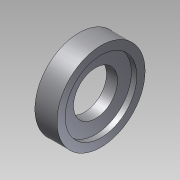
# Autodesk Inventor part: Pusher.springplate
Saved by Autodesk Inventor 2011 (Build 150239000, 239)
## iProperties
Created: 2011-04-01
Part Number: Pusher.springplate
Document SubType Name: Modeling
Designer: Casey
Density: 1 g/cm^3
Author: Casey
Autodesk Inventor part; units mm, degrees
ref_plane "YZ Plane" through (0, 0, 0) normal (1, 0, 0) x (0, 1, 0)
ref_plane "XZ Plane" through (0, 0, 0) normal (0, 1, 0) x (-1, 0, 0)
ref_plane "XY Plane" through (0, 0, 0) normal (0, 0, 1) x (1, 0, 0)
sketch "Sketch1" plane through (0, 0, 0) normal (0, 0, 1) x (1, 0, 0)
  line L0 (0, 2) -> (0.5, 2)
  line L1 (0.5, 2) -> (0.5, 3.25)
  line L2 (0.5, 3.25) -> (1, 3.25)
  line L3 (1, 3.25) -> (1, 4)
  line L4 (1, 4) -> (0, 4)
  line L5 (0, 4) -> (0, 2) construction
  line L6 (0, 0) -> (5.2426, 0) construction
  line L7 (0, 2) -> (-0.5, 2)
  line L8 (-0.5, 2) -> (-0.5, 3.25)
  line L9 (-0.5, 3.25) -> (-1, 3.25)
  line L10 (-1, 3.25) -> (-1, 4)
  line L11 (-1, 4) -> (0, 4)
  dimension "d0" = 4
  dimension "d1" = 0.5
  dimension "d2" = 8
  dimension "d4" = 0.5
  dimension "d5" = 6.5
  constraints: 24 end point, 4 symmetric about line, 3 parallel, 3 perpendicular, 1 horizontal, 1 point on line
  measures "d0" diameter of L0 L6
  measures "d1" distance between parallel lines of L3 L1
  measures "d2" diameter of L4 L6
  measures "d4" distance between parallel lines of L5 L1
  measures "d5" diameter of L2 L6
revolve "Revolution1" add sketch "Sketch1" angle 360 about axis through (0, 0, 0) along (1, 0, 0)
body "Solid1"
